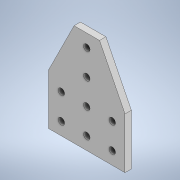
# Autodesk Inventor part: 1x3 t plate
Saved by Autodesk Inventor 2020 (Build 240168000, 168)
## iProperties
Created: 2020-01-14
Part Number: 1x3 t plate
Material: Generic
Document SubType Name: Modeling
Designer: 334334
Density: 1 g/cm^3
Appearance: Default
Author: 334334
Autodesk Inventor part; units mm, degrees
ref_plane "YZ Plane" through (0, 0, 0) normal (1, 0, 0) x (0, 1, 0)
ref_plane "XZ Plane" through (0, 0, 0) normal (0, 1, 0) x (-1, 0, 0)
ref_plane "XY Plane" through (0, 0, 0) normal (0, 0, 1) x (1, 0, 0)
sketch "Sketch1" plane through (0, 0, 0) normal (0, 0, 1) x (1, 0, 0)
  line L0 (0, 0) -> (76.2, 0)
  line L1 (76.2, 0) -> (76.2, 50.8)
  line L2 (0, 50.8) -> (0, 0)
  line L3 (0, 0) -> (50.8, 0)
  line L4 (50.8, 101.6) -> (25.4, 101.6)
  line L5 (0, 50.8) -> (0, 0)
  line L6 (25.4, 101.6) -> (0, 50.8)
  line L7 (50.8, 101.6) -> (76.2, 50.8)
  line L8 (76.2, 50.8) -> (0, 50.8) construction
  circle A0 centre (12.7, 12.7) radius 3.2512
  circle A1 centre (12.7, 38.1) radius 3.2512
  circle A2 centre (38.1, 12.7) radius 3.2512
  circle A3 centre (38.1, 38.1) radius 3.2512
  circle A4 centre (63.5, 12.7) radius 3.2512
  circle A5 centre (63.5, 38.1) radius 3.2512
  circle A6 centre (38.1, 63.5) radius 3.2512
  circle A7 centre (38.1, 88.9) radius 3.2512
  dimension "d10" = 50.8
  dimension "d13" = 76.2
  dimension "d14" = 25.4
  dimension "d15" = 25.4
  dimension "d16" = 50.8
  dimension "d17" = 6.5024
  dimension "d18" = 12.7
  dimension "d19" = 12.7
  dimension "d22" = 25.4
  dimension "d25" = 25.4
  dimension "d30" = 25.4
  constraints: 18 end point, 8 centre point, 5 horizontal, 3 vertical, 2 parallel, 1 perpendicular, 14 other
  measures "d10" distance of L0.end L1.end
  measures "d13" distance of L0.start L0.end
  measures "d14" distance of L4.start L4.end
  measures "d15" horizontal distance of L4.start L1.end
  measures "d16" vertical distance of L4.start L1.end
  measures "d17" diameter of A0
  measures "d18" distance from line of L2 A0.centre
  measures "d19" distance from line of L0 A0.centre
  measures "d22" distance of A0.centre A1.centre
  measures "d25" distance of A0.centre A2.centre
  measures "d30" distance of A3.centre A6.centre
extrude "Extrusion1" add sketch "Sketch1" along normal blind 6.35
body "Solid1"
